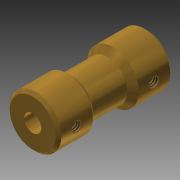
# Autodesk Inventor part: coupler_0305
Saved by Autodesk Inventor 2013 (Build 170138000, 138)
## iProperties
Created: 2015-02-20
Part Number: coupler_0305
Material: 一般
Document SubType Name: Modeling
Designer: Noa Izumi
Density: 1 g/cm^3
Author: Noa Izumi
Autodesk Inventor part; units mm, degrees
ref_plane "YZ Plane" through (0, 0, 0) normal (1, 0, 0) x (0, 1, 0)
ref_plane "XZ Plane" through (0, 0, 0) normal (0, 1, 0) x (-1, 0, 0)
ref_plane "XY Plane" through (0, 0, 0) normal (0, 0, 1) x (1, 0, 0)
sketch "草圖1" plane through (0, 0, 0) normal (0, 1, 0) x (-1, 0, 0)
  circle A0 centre (0, 0) radius 4.5
  dimension "d0" = 9
  constraints: 1 centre point, 1 coincident
  measures "d0" diameter of A0
extrude "擠出1" add sketch "草圖1" along normal blind 6
sketch "草圖2" plane through (0, 6, 0) normal (0, 1, 0) x (1, 0, 0)
  circle A0 centre (0, 0) radius 4.5 projected
  circle A1 centre (0, 0) radius 3.5
  dimension "d4" = 7
  constraints: 1 centre point, 1 coincident
  measures "d4" diameter of A1
extrude "擠出2" add sketch "草圖2" along normal blind 8 contours A1
sketch "草圖3" plane through (0, 14, 0) normal (0, 1, 0) x (1, 0, 0)
  circle A0 centre (0, 0) radius 3.5 projected
  circle A1 centre (0, 0) radius 4.5
  dimension "d8" = 9
  constraints: 1 centre point, 1 coincident
  measures "d8" diameter of A1
extrude "擠出3" add sketch "草圖3" along normal blind 6 contours A0 | A1
chamfer "倒角1" distance 1 angle 45 2 edges at (-3.5, 14, 0) (-3.5, 6, 0)
chamfer "倒角2" distance 0.5 angle 45 2 edges at (-4.5, 20, 0) (4.5, 0, 0)
sketch "草圖4" plane through (0, 0, 0) normal (0, -1, 0) x (1, 0, 0)
  circle A0 centre (0, 0) radius 4 projected
  constraints: 1 coincident
hole "孔1" at (0, 0, 0) direction (0, 1, 0) diameter 3 depth 14 tip angle 118
sketch "草圖5" plane through (0, 20, 0) normal (0, 1, 0) x (1, 0, 0)
  circle A0 centre (0, 0) radius 4 projected
  constraints: 1 coincident
hole "孔2" at (0, 20, 0) direction (0, -1, 0) diameter 5 depth 7 tip angle 118
sketch "草圖6" plane through (0, 0, 0) normal (1, 0, 0) x (0, 1, 0)
  point P0 (0, 0)
  point P1 (3.25, 0)
  point P2 (16.75, 0)
  dimension "d32" = 3.25
  dimension "d33" = 13.5
  measures "d32" distance of point (3.25, 0) point (0, 0)
  measures "d33" distance of point (16.75, 0) point (3.25, 0)
hole "孔3" at (0, 3.25, 0) at (0, 16.75, 0) direction (1, 0, 0) diameter 1.567 end through all thread size "M2x0.4" class "6H" standard "ANSI Metric M Profile"
sketch "草圖7" plane through (0, 0, 0) normal (1, 0, 0) x (0, 1, 0)
  point P0 (0, 0)
  point P1 (3.25, 0)
  point P2 (16.75, 0)
  dimension "d41" = 3.25
  dimension "d42" = 13.5
  measures "d41" distance of point (0, 0) point (3.25, 0)
  measures "d42" distance of point (16.75, 0) point (3.25, 0)
hole "孔4" at (0, 3.25, 0) at (0, 16.75, 0) direction (-1, 0, 0) diameter 1.567 end through all thread size "M2x0.4" class "6H" standard "ANSI Metric M Profile"
chamfer "倒角3" distance 0.125 angle 45 8 edges at (4.4631, 16.2182, 0.5754) (4.4633, 17.2837, 0.5736) (4.4313, 16.7509, -0.7835) (4.4313, 3.2685, -0.7833) (-4.4313, 16.7684, 0.7833) (-4.4631, 2.7181, -0.5753) (-4.4313, 3.2509, 0.7835) (-4.4633, 3.7837, -0.5736)
